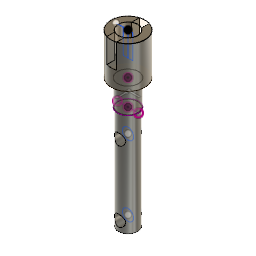
Wheel Cup (Autodesk Fusion 360 design; units mm, degrees)
Autodesk Fusion 360 part; units mm, degrees
sketch "Sketch1" plane through (0, 0, 0) normal (0, 0, 1) x (1, 0, 0)
  circle A0 centre (0, 0) radius 7
  circle A1 centre (0, 0) radius 4
  dimension "d8" = 14
  dimension "d16" = 8
  constraint coincident A0.centre A1.centre
  constraint concentric A0 A1
  measures "d8" diameter of A0
  measures "d16" diameter of A1
extrude "Extrude2" add sketch "Sketch1" against normal blind 17 contours A0 | A1 makes body 1
extrude "Extrude1" add sketch "Sketch1" against normal blind 17 separate body contours A0 | A1 makes body 2
extrude "Extrude3" cut sketch "Sketch1" against normal blind 10 contours A1 bodies 1 2
sketch "Sketch2" plane through (0, 0, 0) normal (0, 1, 0) x (1, 0, 0)
  line L0 (-5, 0) -> (0, 0)
  line L1 (0, 0) -> (-2, 0)
  line L2 (-2, 0) -> (-2, 10)
  line L3 (-2, 10) -> (0, 10)
  line L4 (0, 10) -> (0, 0)
  line L5 (0, 0) -> (2, 0)
  line L6 (2, 0) -> (2, 10)
  line L7 (2, 10) -> (0, 10)
  line L8 (0, 10) -> (0, 0)
  dimension "d23" = 2
  dimension "d24" = 10
  dimension "d25" = 10
  dimension "d26" = 2
  constraint horizontal L0
  constraint horizontal L1
  constraint vertical L2
  constraint horizontal L3
  constraint vertical L4
  constraint horizontal L5
  constraint vertical L6
  constraint horizontal L7
  constraint vertical L8
  measures "d23" distance of L0.end L1.end
  measures "d24" distance of L0.end L3.end
  measures "d25" distance of L0.end L3.end
  measures "d26" distance of L0.end L5.end
extrude "Extrude4" cut sketch "Sketch2" along normal mid plane 200 contours L0 L1 L2 L3 L4 L8 bodies 1 2
extrude "Extrude5" cut sketch "Sketch2" along normal mid plane 200 contours L4 L5 L6 L7 L8 bodies 1 2
sketch "Sketch3" plane through (0, 0, -17) normal (0, 0, -1) x (1, 0, 0)
  circle A0 centre (0, 0) radius 7
  circle A1 centre (0, 0) radius 4.3
  dimension "d31" = 8.6
  constraint coincident A0.centre A1.centre
  measures "d31" diameter of A1
extrude "Extrude6" add sketch "Sketch3" along normal blind 10.5 contours A1 bodies 1 2
sketch "Sketch5" plane through (0, 0, 0) normal (0, 1, 0) x (1, 0, 0)
  circle A0 centre (0, 66) radius 2.3
  line L0 (4.3, 27.5) -> (-4.3, 27.5)
  circle A1 centre (0, 37) radius 2.3
  point P0 (0, 17)
  dimension "d36" = 4.6
  dimension "d40" = 4.6
  dimension "d54" = 20
  dimension "d55" = 29
  measures "d36" diameter of A0
  measures "d40" diameter of A1
  measures "d54" distance of A1.centre P0
  measures "d55" distance of A0.centre A1.centre
extrude "Extrude8" cut sketch "Sketch5" along normal mid plane 200 contours A1 bodies 1
extrude "Extrude7" cut sketch "Sketch5" along normal mid plane 200 contours A0 bodies 1
sketch "Sketch6" plane through (0, 0, -27.5) normal (0, 0, -1) x (1, 0, 0)
  circle A0 centre (0, 0) radius 3.98
  circle A1 centre (0, 0) radius 4.3
  dimension "d47" = 7.96
  constraint coincident A0.centre A1.centre
  measures "d47" diameter of A0
extrude "Extrude9" add sketch "Sketch6" along normal blind 42.5 contours A0 bodies 1
extrude "Extrude10" cut sketch "Sketch5" along normal mid plane 200 contours A1 bodies 1
extrude "Extrude11" cut sketch "Sketch5" along normal mid plane 200 contours A0 bodies 1
equation "inside_part_outer_radius = 7 mm"
equation "inside_part_inner_radius = 4 mm"
equation "inside_part_length = 17 mm"
equation "outside_part_outer_radius = 3.98 mm"
equation "outside_part_length = 42.5 mm"
equation "wheel_hole_distance = 29 mm"
equation "hub_nut_hole_distance = 20 mm"
equation "d8 = inside_part_outer_radius * 2"
equation "dogbone_side_gap_half_width = 2 mm"
equation "extra = 100 mm"
equation "d11 = -inside_part_length"
equation "d14 = -inside_part_length"
equation "d16 = inside_part_inner_radius * 2"
equation "d17 = -dogbone_side_gap_length"
equation "dogbone_side_gap_length = 10 mm"
equation "d23 = dogbone_side_gap_half_width"
equation "d24 = dogbone_side_gap_length"
equation "d25 = dogbone_side_gap_length"
equation "d26 = dogbone_side_gap_half_width"
equation "d27 = extra"
equation "d29 = extra"
equation "d31 = medium_part_outer_radius * 2"
equation "d32 = medium_part_length"
equation "dowel_pin_hole_radius = 2.3 mm"
equation "d36 = dowel_pin_hole_radius * 2"
equation "d37 = extra"
equation "d40 = dowel_pin_hole_radius * 2"
equation "d42 = extra"
equation "medium_part_outer_radius = 4.30 mm"
equation "medium_part_length = 10.5 mm"
equation "d47 = outside_part_outer_radius * 2"
equation "d48 = outside_part_length"
equation "d50 = extra"
equation "d52 = extra"
equation "d54 = hub_nut_hole_distance"
equation "d55 = wheel_hole_distance"
